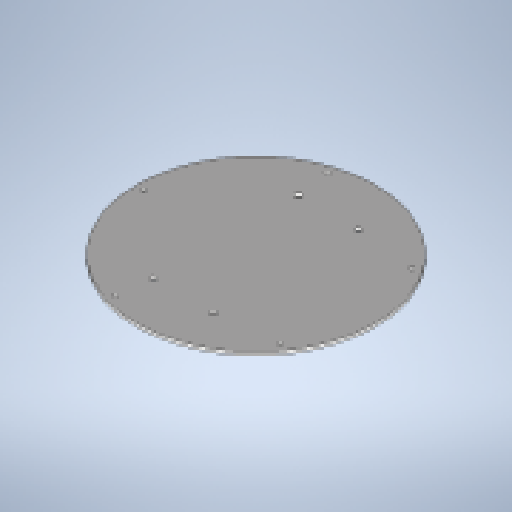
# Autodesk Inventor part: base_plate7
Saved by Autodesk Inventor 2024 (Build 280153000, 153)
## iProperties
Created: 2025-02-22
Part Number: base_plate7
Material: アルミニウム 6061
Document SubType Name: Modeling
Designer: tanoue_kota
Density: 2.7 g/cm^3
Appearance: アルミニウム - フラット
Author: tanoue_kota
Autodesk Inventor part; units mm, degrees
ref_plane "YZ Plane" through (0, 0, 0) normal (1, 0, 0) x (0, 1, 0)
ref_plane "XZ Plane" through (0, 0, 0) normal (0, 1, 0) x (-1, 0, 0)
ref_plane "XY Plane" through (0, 0, 0) normal (0, 0, 1) x (1, 0, 0)
sketch "スケッチ1" plane through (0, 0, 0) normal (0, 1, 0) x (-1, 0, 0)
  circle A0 centre (0, 0) radius 75
  dimension "d0" = 150
  constraints: 1 centre point, 1 coincident
  measures "d0" diameter of A0
extrude "押し出し1" add sketch "スケッチ1" along normal blind 2
sketch "スケッチ2" plane through (0, 2, 0) normal (0, 1, 0) x (1, 0, 0)
  circle A0 centre (0, 0) radius 49
  line L0 (0, 0) -> (0, -49)
  line L1 (0, 0) -> (-18.7515, -45.2701)
  line L2 (0, 0) -> (-49, 0)
  point P0 (18.7515, -45.2701)
  point P1 (-18.7515, 45.2701)
  point P2 (18.7515, 45.2701)
  dimension "d3" = 98
  dimension "d4" = 22.5
  constraints: 6 end point, 3 point on circle, 3 symmetric about line, 2 coincident, 1 centre point, 1 perpendicular, 1 vertical
  measures "d3" diameter of A0
  measures "d4" angle of L0 L1
hole "穴1" at (-18.7515, 2, 45.2701) at (18.7515, 2, 45.2701) at (18.7515, 2, -45.2701) at (-18.7515, 2, -45.2701) direction (0, -1, 0) diameter 4.2 end through all
sketch "スケッチ3" plane through (0, 2, 0) normal (0, 1, 0) x (1, 0, 0)
  circle A0 centre (0, 0) radius 70
  point P0 (-70, 0)
  point P1 (-21.6312, -66.574)
  point P2 (56.6312, -41.145)
  point P3 (56.6312, 41.145)
  point P4 (-21.6312, 66.574)
  dimension "d12" = 140
  dimension "d15" = 360
  constraints: 1 coincident, 1 horizontal alignment, 8 other
hole "穴2" at (-70, 2, 0) at (-21.6312, 2, 66.574) at (56.6312, 2, 41.145) at (56.6312, 2, -41.145) at (-21.6312, 2, -66.574) direction (0, -1, 0) diameter 3.2 end through all
